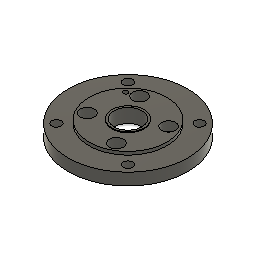
Example (Autodesk Fusion 360 design; units mm, degrees)
Autodesk Fusion 360 part; units mm, degrees
sketch "Sketch1" plane through (0, 0, 0) normal (0, 1, 0) x (1, 0, 0)
  circle A0 centre (0, 0) radius 150
  circle A1 centre (-36.4232, 65.5618) radius 11.5
  circle A2 centre (-36.4232, 65.5618) radius 17.5
  circle A3 centre (-65.5618, -36.4232) radius 17.5
  circle A4 centre (-65.5618, -36.4232) radius 11.5
  circle A5 centre (36.4232, -65.5618) radius 17.5
  circle A6 centre (36.4232, -65.5618) radius 11.5
  circle A7 centre (65.5618, 36.4232) radius 17.5
  circle A8 centre (65.5618, 36.4232) radius 11.5
  circle A9 centre (0, 0) radius 35
  circle A10 centre (0, 0) radius 40.15
  circle A11 centre (0, 0) radius 43.5
  circle A12 centre (0, 0) radius 97.5
  line L0 (0, 0) -> (169.7056, 0) construction
  circle A13 centre (-89.8026, 89.8026) radius 11.75
  circle A14 centre (-89.8026, -89.8026) radius 11.75
  circle A15 centre (89.8026, -89.8026) radius 11.75
  circle A16 centre (89.8026, 89.8026) radius 11.75
  circle A17 centre (-62.8594, 56.9974) radius 6
  dimension "d13" = 300
  dimension "d17" = 23
  dimension "d18" = 35
  dimension "d21" = 70
  dimension "d22" = 80.3
  dimension "d23" = 87
  dimension "d24" = 195
  dimension "d26" = 23.5
  dimension "d28" = 360
  dimension "d31" = 12
  constraint coincident A0.centre A9.centre
  constraint concentric A1 A2
  constraint concentric A0 A9
  constraint concentric A10 A11
  constraint horizontal L0
  measures "d13" diameter of A0
  measures "d17" diameter of A1
  measures "d18" diameter of A2
  measures "d21" diameter of A9
  measures "d22" diameter of A10
  measures "d23" diameter of A11
  measures "d24" diameter of A12
  measures "d26" diameter of A13
  measures "d31" diameter of A17
extrude "Extrude1" add sketch "Sketch1" along normal blind 40 contours A10 makes body 1
extrude "Extrude2" add sketch "Sketch1" along normal blind 38 contours A11 | A12 bodies 1
extrude "Extrude3" add sketch "Sketch1" along normal blind 30 contours A0 bodies 1
extrude "Extrude4" add sketch "Sketch1" along normal blind 5 separate body contours A10 | A11 makes body 2
combine "Combine1" operation cut target body 1 tool bodies 2
extrude "Extrude5" add sketch "Sketch1" along normal blind 14 separate body contours A2 | A3 | A5 | A7 makes body 3 at (83.04, 4.6667, -35.5509) makes body 4 at (-48.0835, 4.6667, 37.2955) makes body 5 at (-18.945, 4.6667, -64.6895) makes body 6 at (53.8363, 9.3333, 67.3042)
combine "Combine2" operation add target body 1 tool bodies 3 5 4 6
scale "Scale1" factor 0.2 about (-35, 5, 0) bodies 1
scale "Scale2" factor 1.5 about (-35, 5, 0) bodies 1
